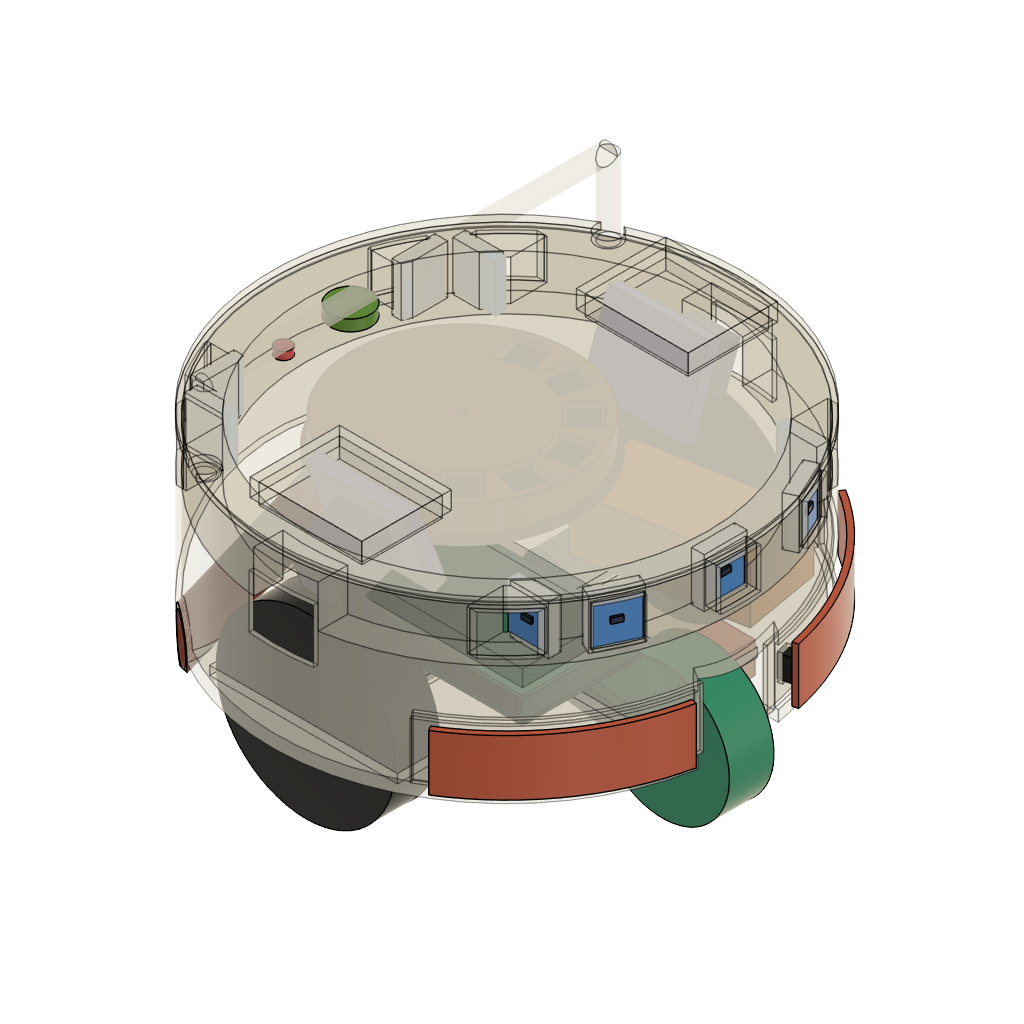
Theseus_V3_baseline (Autodesk Fusion 360 design; units mm, degrees)
Autodesk Fusion 360 part; units mm, degrees
(part 1 of 2)
sketch "Chassis shell sketch" plane through (0, 0, 0) normal (0, 0, 1) x (1, 0, 0) in component "Chassis"
  circle A0 centre (0, 0) radius 105
extrude "Chassis shell" add sketch "Chassis shell sketch" along normal blind 77 from surface at 35 makes body 1 in component "Chassis"
sketch "Cavity sketch" plane through (0, 0, 0) normal (0, 0, 1) x (1, 0, 0) in component "Chassis"
  circle A0 centre (0, 0) radius 103
extrude "Cavity" cut sketch "Cavity sketch" along normal blind 78 from surface at 39 bodies 1 in component "Chassis"
sketch "Rear chamfer sketch" plane through (0, 0, 0) normal (0, 1, 0) x (1, 0, 0) in component "Chassis"
  line L0 (-65, -35) -> (-112, -56.15)
  line L1 (-112, -56.15) -> (-112, -29)
  line L2 (-112, -29) -> (-65, -29)
  line L3 (-65, -29) -> (-65, -35)
extrude "Rear chamfer" cut sketch "Rear chamfer sketch" along normal blind 220 from surface at -110 bodies 1 in component "Chassis"
sketch "Wheel opening L sketch" plane through (0, 0, 0) normal (0, 0, 1) x (1, 0, 0) in component "Chassis"
  line L0 (-42, 69) -> (42, 69)
  line L1 (42, 69) -> (42, 91)
  line L2 (42, 91) -> (-42, 91)
  line L3 (-42, 91) -> (-42, 69)
extrude "Wheel opening L" cut sketch "Wheel opening L sketch" along normal blind 6 from surface at 34 bodies 1 in component "Chassis"
sketch "Motor and shaft slot L sketch" plane through (0, 0, 0) normal (0, 0, 1) x (1, 0, 0) in component "Chassis"
  line L0 (-10.5, 13.5) -> (10.5, 13.5)
  line L1 (10.5, 13.5) -> (10.5, 91)
  line L2 (10.5, 91) -> (-10.5, 91)
  line L3 (-10.5, 91) -> (-10.5, 13.5)
extrude "Motor and shaft slot L" cut sketch "Motor and shaft slot L sketch" along normal blind 6 from surface at 34 bodies 1 in component "Chassis"
sketch "Wheel opening R sketch" plane through (0, 0, 0) normal (0, 0, 1) x (1, 0, 0) in component "Chassis"
  line L0 (-42, -91) -> (42, -91)
  line L1 (42, -91) -> (42, -69)
  line L2 (42, -69) -> (-42, -69)
  line L3 (-42, -69) -> (-42, -91)
extrude "Wheel opening R" cut sketch "Wheel opening R sketch" along normal blind 6 from surface at 34 bodies 1 in component "Chassis"
sketch "Motor and shaft slot R sketch" plane through (0, 0, 0) normal (0, 0, 1) x (1, 0, 0) in component "Chassis"
  line L0 (-10.5, -91) -> (10.5, -91)
  line L1 (10.5, -91) -> (10.5, -13.5)
  line L2 (10.5, -13.5) -> (-10.5, -13.5)
  line L3 (-10.5, -13.5) -> (-10.5, -91)
extrude "Motor and shaft slot R" cut sketch "Motor and shaft slot R sketch" along normal blind 6 from surface at 34 bodies 1 in component "Chassis"
sketch "Omni bay 1 sketch" plane through (0, 0, 0) normal (0, 1, 0) x (1, 0, 0) in component "Chassis"
  line L0 (48.0005, -29.8229) -> (47.9302, -42.3229)
  arc A0 (47.9302, -42.3229) -> (110.9292, -42.6771) centre (79.4297, -42.5) ccw
  line L1 (110.9292, -42.6771) -> (110.9995, -30.1771)
  arc A1 (110.9995, -30.1771) -> (48.0005, -29.8229) centre (79.5, -30) ccw
extrude "Omni bay 1" cut sketch "Omni bay 1 sketch" along normal blind 36 from surface at -18 bodies 1 in component "Chassis"
sketch "Omni bay 2 sketch" plane through (0, 0, 0) normal (0, 1, 0) x (1, 0, 0) in component "Chassis"
  line L0 (49.2548, -33.4597) -> (45.5099, -45.9597)
  arc A0 (45.5099, -45.9597) -> (105.8596, -64.0403) centre (75.6848, -55) ccw
  line L1 (105.8596, -64.0403) -> (109.6046, -51.5403)
  arc A1 (109.6046, -51.5403) -> (49.2548, -33.4597) centre (79.4297, -42.5) ccw
extrude "Omni bay 2" cut sketch "Omni bay 2 sketch" along normal blind 36 from surface at -18 bodies 1 in component "Chassis"
sketch "Arm bay rest sketch" plane through (0, 0, 0) normal (0, 1, 0) x (1, 0, 0) in component "Chassis"
  line L0 (36.069, -43.9283) -> (80.569, -37.9283)
  arc A0 (80.569, -37.9283) -> (78.431, -22.0717) centre (79.5, -30) ccw
  line L1 (78.431, -22.0717) -> (33.931, -28.0717)
  arc A1 (33.931, -28.0717) -> (36.069, -43.9283) centre (35, -36) ccw
extrude "Arm bay rest" cut sketch "Arm bay rest sketch" along normal blind 36 from surface at -18 bodies 1 in component "Chassis"
sketch "Arm bay mid sketch" plane through (0, 0, 0) normal (0, 1, 0) x (1, 0, 0) in component "Chassis"
  line L0 (33.8419, -43.9157) -> (78.2717, -50.4157)
  arc A0 (78.2717, -50.4157) -> (80.5878, -34.5843) centre (79.4297, -42.5) ccw
  line L1 (80.5878, -34.5843) -> (36.1581, -28.0843)
  arc A1 (36.1581, -28.0843) -> (33.8419, -43.9157) centre (35, -36) ccw
extrude "Arm bay mid" cut sketch "Arm bay mid sketch" along normal blind 36 from surface at -18 bodies 1 in component "Chassis"
sketch "Arm bay compressed sketch" plane through (0, 0, 0) normal (0, 1, 0) x (1, 0, 0) in component "Chassis"
  line L0 (31.6149, -43.2485) -> (72.2997, -62.2485)
  arc A0 (72.2997, -62.2485) -> (79.0699, -47.7515) centre (75.6848, -55) ccw
  line L1 (79.0699, -47.7515) -> (38.3851, -28.7515)
  arc A1 (38.3851, -28.7515) -> (31.6149, -43.2485) centre (35, -36) ccw
extrude "Arm bay compressed" cut sketch "Arm bay compressed sketch" along normal blind 36 from surface at -18 bodies 1 in component "Chassis"
sketch "Floor port FP hole sketch" plane through (0, 0, 0) normal (0, 0, 1) x (1, 0, 0) in component "Chassis"
  line L0 (56.5, 21.5) -> (73.5, 21.5)
  line L1 (73.5, 21.5) -> (73.5, 38.5)
  line L2 (73.5, 38.5) -> (56.5, 38.5)
  line L3 (56.5, 38.5) -> (56.5, 21.5)
extrude "Floor port FP hole" cut sketch "Floor port FP hole sketch" along normal blind 6 from surface at 34 bodies 1 in component "Chassis"
sketch "Silver module SM hole sketch" plane through (0, 0, 0) normal (0, 0, 1) x (1, 0, 0) in component "Chassis"
  line L0 (-10.5, -11.5) -> (10.5, -11.5)
  line L1 (10.5, -11.5) -> (10.5, 11.5)
  line L2 (10.5, 11.5) -> (-10.5, 11.5)
  line L3 (-10.5, 11.5) -> (-10.5, -11.5)
extrude "Silver module SM hole" cut sketch "Silver module SM hole sketch" along normal blind 6 from surface at 34 bodies 1 in component "Chassis"
sketch "Chute hole tool B left sketch" plane through (0, 0, 0) normal (0, 0, 1) x (1, 0, 0) in component "Chassis"
  circle A0 centre (0, 0) radius 9
extrude "Chute hole tool B left" add sketch "Chute hole tool B left sketch" along normal blind 78.4275 separate body makes body 2 in component "Chassis"
move_body "Move1" bodies 2 to x (-0.977496, -0.210954, 0) y (-0.120664, 0.559121, 0.820259) z (-0.173037, 0.801799, -0.571993) at (-47.2943, 27.2943, 79.5) in component "Chassis"
combine "Combine1" operation cut target body 1 tool bodies 2 in component "Chassis"
sketch "Chute hole tool A right sketch" plane through (0, 0, 0) normal (0, 0, 1) x (1, 0, 0) in component "Chassis"
  circle A0 centre (0, 0) radius 9
extrude "Chute hole tool A right" add sketch "Chute hole tool A right sketch" along normal blind 78.4275 separate body makes body 3 in component "Chassis"
move_body "Move2" bodies 3 to x (0.977496, -0.210954, 0) y (-0.120664, -0.559121, 0.820259) z (-0.173037, -0.801799, -0.571993) at (-47.2943, -27.2943, 79.5) in component "Chassis"
combine "Combine2" operation cut target body 1 tool bodies 3 in component "Chassis"
sketch "ToF window F sketch" plane through (0, 0, 0) normal (0, 0, 1) x (1, 0, 0) in component "Chassis"
  line L0 (95, 9) -> (108, 9)
  line L1 (108, 9) -> (108, -9)
  line L2 (108, -9) -> (95, -9)
  line L3 (95, -9) -> (95, 9)
extrude "ToF window F" cut sketch "ToF window F sketch" along normal blind 18 from surface at 91 bodies 1 in component "Chassis"
sketch "ToF window FL sketch" plane through (0, 0, 0) normal (0, 0, 1) x (1, 0, 0) in component "Chassis"
  line L0 (85.9209, 49.996) -> (94.0777, 53.7995)
  line L1 (94.0777, 53.7995) -> (101.6848, 37.486)
  line L2 (101.6848, 37.486) -> (93.528, 33.6824)
  line L3 (93.528, 33.6824) -> (85.9209, 49.996)
extrude "ToF window FL" cut sketch "ToF window FL sketch" along normal blind 18 from surface at 91 bodies 1 in component "Chassis"
sketch "ToF window FR sketch" plane through (0, 0, 0) normal (0, 0, 1) x (1, 0, 0) in component "Chassis"
  line L0 (93.528, -33.6824) -> (101.6848, -37.486)
  line L1 (101.6848, -37.486) -> (94.0777, -53.7995)
  line L2 (94.0777, -53.7995) -> (85.9209, -49.996)
  line L3 (85.9209, -49.996) -> (93.528, -33.6824)
extrude "ToF window FR" cut sketch "ToF window FR sketch" along normal blind 18 from surface at 91 bodies 1 in component "Chassis"
sketch "ToF window SFL sketch" plane through (0, 0, 0) normal (0, 0, 1) x (1, 0, 0) in component "Chassis"
  line L0 (62.8, 60) -> (62.8, 80.6769)
  line L1 (62.8, 80.6769) -> (80.8, 80.6769)
  line L2 (80.8, 80.6769) -> (80.8, 60)
  line L3 (80.8, 60) -> (62.8, 60)
extrude "ToF window SFL" cut sketch "ToF window SFL sketch" along normal blind 18 from surface at 91 bodies 1 in component "Chassis"
sketch "ToF window SFR sketch" plane through (0, 0, 0) normal (0, 0, 1) x (1, 0, 0) in component "Chassis"
  line L0 (80.8, -60) -> (80.8, -80.6769)
  line L1 (80.8, -80.6769) -> (62.8, -80.6769)
  line L2 (62.8, -80.6769) -> (62.8, -60)
  line L3 (62.8, -60) -> (80.8, -60)
extrude "ToF window SFR" cut sketch "ToF window SFR sketch" along normal blind 18 from surface at 91 bodies 1 in component "Chassis"
sketch "ToF window SRL sketch" plane through (0, 0, 0) normal (0, 0, 1) x (1, 0, 0) in component "Chassis"
  line L0 (-80.8, 60) -> (-80.8, 80.6769)
  line L1 (-80.8, 80.6769) -> (-62.8, 80.6769)
  line L2 (-62.8, 80.6769) -> (-62.8, 60)
  line L3 (-62.8, 60) -> (-80.8, 60)
extrude "ToF window SRL" cut sketch "ToF window SRL sketch" along normal blind 18 from surface at 91 bodies 1 in component "Chassis"
sketch "ToF window SRR sketch" plane through (0, 0, 0) normal (0, 0, 1) x (1, 0, 0) in component "Chassis"
  line L0 (-62.8, -60) -> (-62.8, -80.6769)
  line L1 (-62.8, -80.6769) -> (-80.8, -80.6769)
  line L2 (-80.8, -80.6769) -> (-80.8, -60)
  line L3 (-80.8, -60) -> (-62.8, -60)
extrude "ToF window SRR" cut sketch "ToF window SRR sketch" along normal blind 18 from surface at 91 bodies 1 in component "Chassis"
sketch "ToF window RL sketch" plane through (0, 0, 0) normal (0, 0, 1) x (1, 0, 0) in component "Chassis"
  line L0 (-84, 36) -> (-98.1784, 36)
  line L1 (-98.1784, 36) -> (-98.1784, 54)
  line L2 (-98.1784, 54) -> (-84, 54)
  line L3 (-84, 54) -> (-84, 36)
extrude "ToF window RL" cut sketch "ToF window RL sketch" along normal blind 18 from surface at 91 bodies 1 in component "Chassis"
sketch "ToF window RR sketch" plane through (0, 0, 0) normal (0, 0, 1) x (1, 0, 0) in component "Chassis"
  line L0 (-84, -54) -> (-98.1784, -54)
  line L1 (-98.1784, -54) -> (-98.1784, -36)
  line L2 (-98.1784, -36) -> (-84, -36)
  line L3 (-84, -36) -> (-84, -54)
extrude "ToF window RR" cut sketch "ToF window RR sketch" along normal blind 18 from surface at 91 bodies 1 in component "Chassis"
sketch "Camera window L sketch" plane through (0, 0, 0) normal (0, 1, 0) x (1, 0, 0) in component "Chassis"
  line L0 (-10.9288, -74) -> (17.0712, -74)
  line L1 (17.0712, -74) -> (17.0712, -98)
  line L2 (17.0712, -98) -> (-10.9288, -98)
  line L3 (-10.9288, -98) -> (-10.9288, -74)
extrude "Camera window L" cut sketch "Camera window L sketch" along normal blind 19 from surface at 89 bodies 1 in component "Chassis"
sketch "Camera window R sketch" plane through (0, 0, 0) normal (0, 1, 0) x (1, 0, 0) in component "Chassis"
  line L0 (-10.9288, -74) -> (17.0712, -74)
  line L1 (17.0712, -74) -> (17.0712, -98)
  line L2 (17.0712, -98) -> (-10.9288, -98)
  line L3 (-10.9288, -98) -> (-10.9288, -74)
extrude "Camera window R" cut sketch "Camera window R sketch" along normal blind 19 from surface at -108 bodies 1 in component "Chassis"
sketch "Bumper recess L sketch" plane through (0, 0, 0) normal (0, 0, 1) x (1, 0, 0) in component "Chassis"
  arc A0 (106.949, 15.0307) -> (50.7029, 95.3583) centre (0, 0) ccw
  line L0 (50.7029, 95.3583) -> (48.5903, 91.3851)
  arc A1 (102.4927, 14.4044) -> (48.5903, 91.3851) centre (0, 0) ccw
  line L1 (102.4927, 14.4044) -> (106.949, 15.0307)
extrude "Bumper recess L" cut sketch "Bumper recess L sketch" along normal blind 25 from surface at 40 bodies 1 in component "Chassis"
sketch "Bumper recess wall L sketch" plane through (0, 0, 0) normal (0, 0, 1) x (1, 0, 0) in component "Chassis"
  arc A0 (102.1957, 14.3627) -> (48.4495, 91.1202) centre (0, 0) ccw
  line L0 (48.4495, 91.1202) -> (47.6514, 89.6192)
  arc A1 (100.5122, 14.1261) -> (47.6514, 89.6192) centre (0, 0) ccw
  line L1 (100.5122, 14.1261) -> (102.1957, 14.3627)
extrude "Bumper recess wall L" add sketch "Bumper recess wall L sketch" along normal blind 27 from surface at 39 bodies 1 in component "Chassis"
sketch "Bumper switch pocket L sketch" plane through (0, 0, 0) normal (0, 0, 1) x (1, 0, 0) in component "Chassis"
  line L0 (98.18, 21.6448) -> (101.576, 22.4916)
  line L1 (101.576, 22.4916) -> (100.2455, 27.8282)
  line L2 (100.2455, 27.8282) -> (96.8494, 26.9815)
  line L3 (96.8494, 26.9815) -> (98.18, 21.6448)
extrude "Bumper switch pocket L" cut sketch "Bumper switch pocket L sketch" along normal blind 12 from surface at 46.5 bodies 1 in component "Chassis"
sketch "Bumper recess R sketch" plane through (0, 0, 0) normal (0, 0, 1) x (1, 0, 0) in component "Chassis"
  arc A0 (50.7029, -95.3583) -> (106.949, -15.0307) centre (0, 0) ccw
  line L0 (106.949, -15.0307) -> (102.4927, -14.4044)
  arc A1 (48.5903, -91.3851) -> (102.4927, -14.4044) centre (0, 0) ccw
  line L1 (48.5903, -91.3851) -> (50.7029, -95.3583)
extrude "Bumper recess R" cut sketch "Bumper recess R sketch" along normal blind 25 from surface at 40 bodies 1 in component "Chassis"
sketch "Bumper recess wall R sketch" plane through (0, 0, 0) normal (0, 0, 1) x (1, 0, 0) in component "Chassis"
  arc A0 (48.4495, -91.1202) -> (102.1957, -14.3627) centre (0, 0) ccw
  line L0 (102.1957, -14.3627) -> (100.5122, -14.1261)
  arc A1 (47.6514, -89.6192) -> (100.5122, -14.1261) centre (0, 0) ccw
  line L1 (47.6514, -89.6192) -> (48.4495, -91.1202)
extrude "Bumper recess wall R" add sketch "Bumper recess wall R sketch" along normal blind 27 from surface at 39 bodies 1 in component "Chassis"
sketch "Bumper switch pocket R sketch" plane through (0, 0, 0) normal (0, 0, 1) x (1, 0, 0) in component "Chassis"
  line L0 (96.8494, -26.9815) -> (100.2455, -27.8282)
  line L1 (100.2455, -27.8282) -> (101.576, -22.4916)
  line L2 (101.576, -22.4916) -> (98.18, -21.6448)
  line L3 (98.18, -21.6448) -> (96.8494, -26.9815)
extrude "Bumper switch pocket R" cut sketch "Bumper switch pocket R sketch" along normal blind 12 from surface at 46.5 bodies 1 in component "Chassis"
sketch "Handle post L sketch" plane through (0, 0, 0) normal (0, 0, 1) x (1, 0, 0) in component "Chassis"
  circle A0 centre (-45, 90.4) radius 4
extrude "Handle post L" add sketch "Handle post L sketch" along normal blind 34.5 from surface at 111.5 bodies 1 in component "Chassis"
sketch "Handle post R sketch" plane through (0, 0, 0) normal (0, 0, 1) x (1, 0, 0) in component "Chassis"
  circle A0 centre (-45, -90.4) radius 4
extrude "Handle post R" add sketch "Handle post R sketch" along normal blind 34.5 from surface at 111.5 bodies 1 in component "Chassis"
sketch "Handle bar sketch" plane through (0, 0, 0) normal (0, 1, 0) x (1, 0, 0) in component "Chassis"
  circle A0 centre (-45, -146) radius 4
extrude "Handle bar" add sketch "Handle bar sketch" along normal blind 180.8 from surface at -90.4 bodies 1 in component "Chassis"
sketch "Wheel L sketch" plane through (0, 0, 0) normal (0, 1, 0) x (1, 0, 0) in component "Wheel L"
  circle A0 centre (0, -40) radius 40
extrude "Wheel L" add sketch "Wheel L sketch" along normal blind 20 from surface at 70 separate body makes body 4 in component "Wheel L"
sketch "Shaft bore sketch" plane through (0, 0, 0) normal (0, 1, 0) x (1, 0, 0) in component "Wheel L"
  circle A0 centre (0, -40) radius 1.5
extrude "Shaft bore" cut sketch "Shaft bore sketch" along normal blind 22 from surface at 69 bodies 4 in component "Wheel L"
sketch "Encoder L sketch" plane through (0, 0, 0) normal (0, 1, 0) x (1, 0, 0) in component "Motor L"
  circle A0 centre (0, -40) radius 9
extrude "Encoder L" add sketch "Encoder L sketch" along normal blind 3 from surface at 14 separate body makes body 5 in component "Motor L"
sketch "Gearmotor L sketch" plane through (0, 0, 0) normal (0, 1, 0) x (1, 0, 0) in component "Motor L"
  circle A0 centre (0, -40) radius 10
extrude "Gearmotor L" add sketch "Gearmotor L sketch" along normal blind 44 from surface at 17 separate body makes body 6 in component "Motor L"
sketch "Motor shaft L sketch" plane through (0, 0, 0) normal (0, 1, 0) x (1, 0, 0) in component "Motor L"
  circle A0 centre (0, -40) radius 1.5
extrude "Motor shaft L" add sketch "Motor shaft L sketch" along normal blind 19 from surface at 61 separate body makes body 7 in component "Motor L"
sketch "Wheel R sketch" plane through (0, 0, 0) normal (0, 1, 0) x (1, 0, 0) in component "Wheel R"
  circle A0 centre (0, -40) radius 40
extrude "Wheel R" add sketch "Wheel R sketch" along normal blind 20 from surface at -90 separate body makes body 8 in component "Wheel R"
sketch "Shaft bore sketch (2)" plane through (0, 0, 0) normal (0, 1, 0) x (1, 0, 0) in component "Wheel R"
  circle A0 centre (0, -40) radius 1.5
extrude "Shaft bore'" cut sketch "Shaft bore sketch (2)" along normal blind 22 from surface at -91 bodies 8 in component "Wheel R"
sketch "Encoder R sketch" plane through (0, 0, 0) normal (0, 1, 0) x (1, 0, 0) in component "Motor R"
  circle A0 centre (0, -40) radius 9
extrude "Encoder R" add sketch "Encoder R sketch" along normal blind 3 from surface at -17 separate body makes body 9 in component "Motor R"
sketch "Gearmotor R sketch" plane through (0, 0, 0) normal (0, 1, 0) x (1, 0, 0) in component "Motor R"
  circle A0 centre (0, -40) radius 10
extrude "Gearmotor R" add sketch "Gearmotor R sketch" along normal blind 44 from surface at -61 separate body makes body 10 in component "Motor R"
sketch "Motor shaft R sketch" plane through (0, 0, 0) normal (0, 1, 0) x (1, 0, 0) in component "Motor R"
  circle A0 centre (0, -40) radius 1.5
extrude "Motor shaft R" add sketch "Motor shaft R sketch" along normal blind 19 from surface at -80 separate body makes body 11 in component "Motor R"
sketch "Omni wheel sketch" plane through (0, 0, 0) normal (0, 1, 0) x (1, 0, 0) in component "Omni wheel"
  circle A0 centre (79.5, -30) radius 30
extrude "Omni wheel" add sketch "Omni wheel sketch" along normal blind 20 from surface at -10 separate body makes body 12 in component "Omni wheel"
sketch "Omni hub sketch" plane through (0, 0, 0) normal (0, 1, 0) x (1, 0, 0) in component "Omni wheel"
  circle A0 centre (79.5, -30) radius 10
extrude "Omni hub" add sketch "Omni hub sketch" along normal blind 22 from surface at -11 bodies 12 in component "Omni wheel"
sketch "Axle bore sketch" plane through (0, 0, 0) normal (0, 1, 0) x (1, 0, 0) in component "Omni wheel"
  circle A0 centre (79.5, -30) radius 2
extrude "Axle bore" cut sketch "Axle bore sketch" along normal blind 24 from surface at -12 bodies 12 in component "Omni wheel"
sketch "Arm plate L sketch" plane through (0, 0, 0) normal (0, 1, 0) x (1, 0, 0) in component "Omni arm"
  line L0 (35.7349, -41.4507) -> (80.2349, -35.4507)
  arc A0 (80.2349, -35.4507) -> (78.7651, -24.5493) centre (79.5, -30) ccw
  line L1 (78.7651, -24.5493) -> (34.2651, -30.5493)
  arc A1 (34.2651, -30.5493) -> (35.7349, -41.4507) centre (35, -36) ccw
extrude "Arm plate L" add sketch "Arm plate L sketch" along normal blind 4 from surface at 11 separate body makes body 13 in component "Omni arm"
sketch "Pivot hole L sketch" plane through (0, 0, 0) normal (0, 1, 0) x (1, 0, 0) in component "Omni arm"
  circle A0 centre (35, -36) radius 2
extrude "Pivot hole L" cut sketch "Pivot hole L sketch" along normal blind 6 from surface at 10 bodies 13 in component "Omni arm"
sketch "Axle hole L sketch" plane through (0, 0, 0) normal (0, 1, 0) x (1, 0, 0) in component "Omni arm"
  circle A0 centre (79.5, -30) radius 2
extrude "Axle hole L" cut sketch "Axle hole L sketch" along normal blind 6 from surface at 10 bodies 13 in component "Omni arm"
sketch "Arm plate R sketch" plane through (0, 0, 0) normal (0, 1, 0) x (1, 0, 0) in component "Omni arm"
  line L0 (35.7349, -41.4507) -> (80.2349, -35.4507)
  arc A0 (80.2349, -35.4507) -> (78.7651, -24.5493) centre (79.5, -30) ccw
  line L1 (78.7651, -24.5493) -> (34.2651, -30.5493)
  arc A1 (34.2651, -30.5493) -> (35.7349, -41.4507) centre (35, -36) ccw
extrude "Arm plate R" add sketch "Arm plate R sketch" along normal blind 4 from surface at -15 separate body makes body 14 in component "Omni arm"
sketch "Pivot hole R sketch" plane through (0, 0, 0) normal (0, 1, 0) x (1, 0, 0) in component "Omni arm"
  circle A0 centre (35, -36) radius 2
extrude "Pivot hole R" cut sketch "Pivot hole R sketch" along normal blind 6 from surface at -16 bodies 14 in component "Omni arm"
sketch "Axle hole R sketch" plane through (0, 0, 0) normal (0, 1, 0) x (1, 0, 0) in component "Omni arm"
  circle A0 centre (79.5, -30) radius 2
extrude "Axle hole R" cut sketch "Axle hole R sketch" along normal blind 6 from surface at -16 bodies 14 in component "Omni arm"
sketch "Pivot pin sketch" plane through (0, 0, 0) normal (0, 1, 0) x (1, 0, 0) in component "Omni pins"
  circle A0 centre (35, -36) radius 2
extrude "Pivot pin" add sketch "Pivot pin sketch" along normal blind 34 from surface at -17 separate body makes body 15 in component "Omni pins"
sketch "Axle pin sketch" plane through (0, 0, 0) normal (0, 1, 0) x (1, 0, 0) in component "Omni pins"
  circle A0 centre (79.5, -30) radius 2
extrude "Axle pin" add sketch "Axle pin sketch" along normal blind 30 from surface at -15 separate body makes body 16 in component "Omni pins"
sketch "Rear nub sketch" plane through (0, 0, 0) normal (0, 0, 1) x (1, 0, 0) in component "Rear nub"
  circle A0 centre (-80, 0) radius 4
extrude "Rear nub" add sketch "Rear nub sketch" along normal blind 26 from surface at 20 separate body makes body 17 in component "Rear nub"
sketch "Seat on chamfer sketch" plane through (0, 0, 0) normal (0, 1, 0) x (1, 0, 0) in component "Rear nub"
  line L0 (-65, -35) -> (-112, -56.15)
  line L1 (-112, -56.15) -> (-112, -70)
  line L2 (-112, -70) -> (-65, -70)
  line L3 (-65, -70) -> (-65, -35)
extrude "Seat on chamfer" cut sketch "Seat on chamfer sketch" along normal blind 20 from surface at -10 bodies 17 in component "Rear nub"
sketch "Bumper plate L sketch" plane through (0, 0, 0) normal (0, 0, 1) x (1, 0, 0) in component "Bumper L"
  arc A0 (107.5962, 22.8703) -> (58.2911, 93.2853) centre (0, 0) ccw
  line L0 (58.2911, 93.2853) -> (56.9663, 91.1652)
  arc A1 (105.1509, 22.3505) -> (56.9663, 91.1652) centre (0, 0) ccw
  line L1 (105.1509, 22.3505) -> (107.5962, 22.8703)
extrude "Bumper plate L" add sketch "Bumper plate L sketch" along normal blind 25 from surface at 40 separate body makes body 18 in component "Bumper L"
sketch "Microswitch L sketch" plane through (0, 0, 0) normal (0, 0, 1) x (1, 0, 0) in component "Bumper switch L"
  line L0 (98.5442, 22.2509) -> (104.8511, 23.8234)
  line L1 (104.8511, 23.8234) -> (103.7625, 28.1898)
  line L2 (103.7625, 28.1898) -> (97.4555, 26.6173)
  line L3 (97.4555, 26.6173) -> (98.5442, 22.2509)
extrude "Microswitch L" add sketch "Microswitch L sketch" along normal blind 10 from surface at 47.5 separate body makes body 19 in component "Bumper switch L"
sketch "Bumper plate R sketch" plane through (0, 0, 0) normal (0, 0, 1) x (1, 0, 0) in component "Bumper R"
  arc A0 (58.2911, -93.2853) -> (107.5962, -22.8703) centre (0, 0) ccw
  line L0 (107.5962, -22.8703) -> (105.1509, -22.3505)
  arc A1 (56.9663, -91.1652) -> (105.1509, -22.3505) centre (0, 0) ccw
  line L1 (56.9663, -91.1652) -> (58.2911, -93.2853)
extrude "Bumper plate R" add sketch "Bumper plate R sketch" along normal blind 25 from surface at 40 separate body makes body 20 in component "Bumper R"
sketch "Microswitch R sketch" plane through (0, 0, 0) normal (0, 0, 1) x (1, 0, 0) in component "Bumper switch R"
  line L0 (97.4555, -26.6173) -> (103.7625, -28.1898)
  line L1 (103.7625, -28.1898) -> (104.8511, -23.8234)
  line L2 (104.8511, -23.8234) -> (98.5442, -22.2509)
  line L3 (98.5442, -22.2509) -> (97.4555, -26.6173)
extrude "Microswitch R" add sketch "Microswitch R sketch" along normal blind 10 from surface at 47.5 separate body makes body 21 in component "Bumper switch R"
sketch "ToF ring sketch" plane through (0, 0, 0) normal (0, 0, 1) x (1, 0, 0) in component "ToF ring"
  circle A0 centre (0, 0) radius 103
  circle A1 centre (0, 0) radius 90
extrude "ToF ring" add sketch "ToF ring sketch" along normal blind 24.5 from surface at 87 separate body makes body 22 in component "ToF ring"
sketch "Pocket F sketch" plane through (0, 0, 0) normal (0, 0, 1) x (1, 0, 0) in component "ToF ring"
  line L0 (92.15, 9.6) -> (97.85, 9.6)
  line L1 (97.85, 9.6) -> (97.85, -9.6)
  line L2 (97.85, -9.6) -> (92.15, -9.6)
  line L3 (92.15, -9.6) -> (92.15, 9.6)
extrude "Pocket F" cut sketch "Pocket F sketch" along normal blind 22 from surface at 89 bodies 22 in component "ToF ring"
sketch "Beam F sketch" plane through (0, 0, 0) normal (0, 0, 1) x (1, 0, 0) in component "ToF ring"
  line L0 (95, 9) -> (108, 9)
  line L1 (108, 9) -> (108, -9)
  line L2 (108, -9) -> (95, -9)
  line L3 (95, -9) -> (95, 9)
extrude "Beam F" cut sketch "Beam F sketch" along normal blind 18 from surface at 91 bodies 22 in component "ToF ring"
sketch "Pocket FL sketch" plane through (0, 0, 0) normal (0, 0, 1) x (1, 0, 0) in component "ToF ring"
  line L0 (83.0844, 49.3353) -> (88.2503, 51.7442)
  line L1 (88.2503, 51.7442) -> (96.3646, 34.3431)
  line L2 (96.3646, 34.3431) -> (91.1986, 31.9342)
  line L3 (91.1986, 31.9342) -> (83.0844, 49.3353)
extrude "Pocket FL" cut sketch "Pocket FL sketch" along normal blind 22 from surface at 89 bodies 22 in component "ToF ring"
sketch "Beam FL sketch" plane through (0, 0, 0) normal (0, 0, 1) x (1, 0, 0) in component "ToF ring"
  line L0 (85.9209, 49.996) -> (94.0777, 53.7995)
  line L1 (94.0777, 53.7995) -> (101.6848, 37.486)
  line L2 (101.6848, 37.486) -> (93.528, 33.6824)
  line L3 (93.528, 33.6824) -> (85.9209, 49.996)
extrude "Beam FL" cut sketch "Beam FL sketch" along normal blind 18 from surface at 91 bodies 22 in component "ToF ring"
sketch "Pocket FR sketch" plane through (0, 0, 0) normal (0, 0, 1) x (1, 0, 0) in component "ToF ring"
  line L0 (91.1986, -31.9342) -> (96.3646, -34.3431)
  line L1 (96.3646, -34.3431) -> (88.2503, -51.7442)
  line L2 (88.2503, -51.7442) -> (83.0844, -49.3353)
  line L3 (83.0844, -49.3353) -> (91.1986, -31.9342)
extrude "Pocket FR" cut sketch "Pocket FR sketch" along normal blind 22 from surface at 89 bodies 22 in component "ToF ring"
sketch "Beam FR sketch" plane through (0, 0, 0) normal (0, 0, 1) x (1, 0, 0) in component "ToF ring"
  line L0 (93.528, -33.6824) -> (101.6848, -37.486)
  line L1 (101.6848, -37.486) -> (94.0777, -53.7995)
  line L2 (94.0777, -53.7995) -> (85.9209, -49.996)
  line L3 (85.9209, -49.996) -> (93.528, -33.6824)
extrude "Beam FR" cut sketch "Beam FR sketch" along normal blind 18 from surface at 91 bodies 22 in component "ToF ring"
sketch "Pocket SFL sketch" plane through (0, 0, 0) normal (0, 0, 1) x (1, 0, 0) in component "ToF ring"
  line L0 (62.2, 57.15) -> (62.2, 62.85)
  line L1 (62.2, 62.85) -> (81.4, 62.85)
  line L2 (81.4, 62.85) -> (81.4, 57.15)
  line L3 (81.4, 57.15) -> (62.2, 57.15)
extrude "Pocket SFL" cut sketch "Pocket SFL sketch" along normal blind 22 from surface at 89 bodies 22 in component "ToF ring"
sketch "Beam SFL sketch" plane through (0, 0, 0) normal (0, 0, 1) x (1, 0, 0) in component "ToF ring"
  line L0 (62.8, 60) -> (62.8, 80.6769)
  line L1 (62.8, 80.6769) -> (80.8, 80.6769)
  line L2 (80.8, 80.6769) -> (80.8, 60)
  line L3 (80.8, 60) -> (62.8, 60)
extrude "Beam SFL" cut sketch "Beam SFL sketch" along normal blind 18 from surface at 91 bodies 22 in component "ToF ring"
sketch "Pocket SFR sketch" plane through (0, 0, 0) normal (0, 0, 1) x (1, 0, 0) in component "ToF ring"
  line L0 (81.4, -57.15) -> (81.4, -62.85)
  line L1 (81.4, -62.85) -> (62.2, -62.85)
  line L2 (62.2, -62.85) -> (62.2, -57.15)
  line L3 (62.2, -57.15) -> (81.4, -57.15)
extrude "Pocket SFR" cut sketch "Pocket SFR sketch" along normal blind 22 from surface at 89 bodies 22 in component "ToF ring"
sketch "Beam SFR sketch" plane through (0, 0, 0) normal (0, 0, 1) x (1, 0, 0) in component "ToF ring"
  line L0 (80.8, -60) -> (80.8, -80.6769)
  line L1 (80.8, -80.6769) -> (62.8, -80.6769)
  line L2 (62.8, -80.6769) -> (62.8, -60)
  line L3 (62.8, -60) -> (80.8, -60)
extrude "Beam SFR" cut sketch "Beam SFR sketch" along normal blind 18 from surface at 91 bodies 22 in component "ToF ring"
sketch "Pocket SRL sketch" plane through (0, 0, 0) normal (0, 0, 1) x (1, 0, 0) in component "ToF ring"
  line L0 (-81.4, 57.15) -> (-81.4, 62.85)
  line L1 (-81.4, 62.85) -> (-62.2, 62.85)
  line L2 (-62.2, 62.85) -> (-62.2, 57.15)
  line L3 (-62.2, 57.15) -> (-81.4, 57.15)
extrude "Pocket SRL" cut sketch "Pocket SRL sketch" along normal blind 22 from surface at 89 bodies 22 in component "ToF ring"
sketch "Beam SRL sketch" plane through (0, 0, 0) normal (0, 0, 1) x (1, 0, 0) in component "ToF ring"
  line L0 (-80.8, 60) -> (-80.8, 80.6769)
  line L1 (-80.8, 80.6769) -> (-62.8, 80.6769)
  line L2 (-62.8, 80.6769) -> (-62.8, 60)
  line L3 (-62.8, 60) -> (-80.8, 60)
extrude "Beam SRL" cut sketch "Beam SRL sketch" along normal blind 18 from surface at 91 bodies 22 in component "ToF ring"
sketch "Pocket SRR sketch" plane through (0, 0, 0) normal (0, 0, 1) x (1, 0, 0) in component "ToF ring"
  line L0 (-62.2, -57.15) -> (-62.2, -62.85)
  line L1 (-62.2, -62.85) -> (-81.4, -62.85)
  line L2 (-81.4, -62.85) -> (-81.4, -57.15)
  line L3 (-81.4, -57.15) -> (-62.2, -57.15)
extrude "Pocket SRR" cut sketch "Pocket SRR sketch" along normal blind 22 from surface at 89 bodies 22 in component "ToF ring"
sketch "Beam SRR sketch" plane through (0, 0, 0) normal (0, 0, 1) x (1, 0, 0) in component "ToF ring"
  line L0 (-62.8, -60) -> (-62.8, -80.6769)
  line L1 (-62.8, -80.6769) -> (-80.8, -80.6769)
  line L2 (-80.8, -80.6769) -> (-80.8, -60)
  line L3 (-80.8, -60) -> (-62.8, -60)
extrude "Beam SRR" cut sketch "Beam SRR sketch" along normal blind 18 from surface at 91 bodies 22 in component "ToF ring"
sketch "Pocket RL sketch" plane through (0, 0, 0) normal (0, 0, 1) x (1, 0, 0) in component "ToF ring"
  line L0 (-81.15, 35.4) -> (-86.85, 35.4)
  line L1 (-86.85, 35.4) -> (-86.85, 54.6)
  line L2 (-86.85, 54.6) -> (-81.15, 54.6)
  line L3 (-81.15, 54.6) -> (-81.15, 35.4)
extrude "Pocket RL" cut sketch "Pocket RL sketch" along normal blind 22 from surface at 89 bodies 22 in component "ToF ring"
sketch "Beam RL sketch" plane through (0, 0, 0) normal (0, 0, 1) x (1, 0, 0) in component "ToF ring"
  line L0 (-84, 36) -> (-98.1784, 36)
  line L1 (-98.1784, 36) -> (-98.1784, 54)
  line L2 (-98.1784, 54) -> (-84, 54)
  line L3 (-84, 54) -> (-84, 36)
extrude "Beam RL" cut sketch "Beam RL sketch" along normal blind 18 from surface at 91 bodies 22 in component "ToF ring"
sketch "Pocket RR sketch" plane through (0, 0, 0) normal (0, 0, 1) x (1, 0, 0) in component "ToF ring"
  line L0 (-81.15, -54.6) -> (-86.85, -54.6)
  line L1 (-86.85, -54.6) -> (-86.85, -35.4)
  line L2 (-86.85, -35.4) -> (-81.15, -35.4)
  line L3 (-81.15, -35.4) -> (-81.15, -54.6)
extrude "Pocket RR" cut sketch "Pocket RR sketch" along normal blind 22 from surface at 89 bodies 22 in component "ToF ring"
sketch "Beam RR sketch" plane through (0, 0, 0) normal (0, 0, 1) x (1, 0, 0) in component "ToF ring"
  line L0 (-84, -54) -> (-98.1784, -54)
  line L1 (-98.1784, -54) -> (-98.1784, -36)
  line L2 (-98.1784, -36) -> (-84, -36)
  line L3 (-84, -36) -> (-84, -54)
extrude "Beam RR" cut sketch "Beam RR sketch" along normal blind 18 from surface at 91 bodies 22 in component "ToF ring"
sketch "Camera window L sketch (2)" plane through (0, 0, 0) normal (0, 1, 0) x (1, 0, 0) in component "ToF ring"
  line L0 (-10.9288, -86) -> (17.0712, -86)
  line L1 (17.0712, -86) -> (17.0712, -106)
  line L2 (17.0712, -106) -> (-10.9288, -106)
  line L3 (-10.9288, -106) -> (-10.9288, -86)
extrude "Camera window L'" cut sketch "Camera window L sketch (2)" along normal blind 24 from surface at 84 bodies 22 in component "ToF ring"
sketch "Camera window R sketch (2)" plane through (0, 0, 0) normal (0, 1, 0) x (1, 0, 0) in component "ToF ring"
  line L0 (-10.9288, -86) -> (17.0712, -86)
  line L1 (17.0712, -86) -> (17.0712, -106)
  line L2 (17.0712, -106) -> (-10.9288, -106)
  line L3 (-10.9288, -106) -> (-10.9288, -86)
extrude "Camera window R'" cut sketch "Camera window R sketch (2)" along normal blind 24 from surface at -108 bodies 22 in component "ToF ring"
sketch "VL53L0X module F sketch" plane through (0, 0, 0) normal (0, 0, 1) x (1, 0, 0) in component "ToF F"
  line L0 (92.75, -9) -> (97.25, -9)
  line L1 (97.25, -9) -> (97.25, 9)
  line L2 (97.25, 9) -> (92.75, 9)
  line L3 (92.75, 9) -> (92.75, -9)
extrude "VL53L0X module F" add sketch "VL53L0X module F sketch" along normal blind 21 from surface at 89.5 separate body makes body 23 in component "ToF F"
sketch "VL53L0X chip F sketch" plane through (0, 0, 0) normal (0, 0, 1) x (1, 0, 0) in component "ToF F"
  line L0 (97.25, -2.2) -> (98.25, -2.2)
  line L1 (98.25, -2.2) -> (98.25, 2.2)
  line L2 (98.25, 2.2) -> (97.25, 2.2)
  line L3 (97.25, 2.2) -> (97.25, -2.2)
extrude "VL53L0X chip F" add sketch "VL53L0X chip F sketch" along normal blind 2.4 from surface at 98.8 separate body makes body 24 in component "ToF F"
sketch "VL53L0X module FL sketch" plane through (0, 0, 0) normal (0, 0, 1) x (1, 0, 0) in component "ToF FL"
  line L0 (91.4888, 32.7315) -> (95.5672, 34.6333)
  line L1 (95.5672, 34.6333) -> (87.9601, 50.9469)
  line L2 (87.9601, 50.9469) -> (83.8817, 49.0451)
  line L3 (83.8817, 49.0451) -> (91.4888, 32.7315)
extrude "VL53L0X module FL" add sketch "VL53L0X module FL sketch" along normal blind 21 from surface at 89.5 separate body makes body 25 in component "ToF FL"
sketch "VL53L0X chip FL sketch" plane through (0, 0, 0) normal (0, 0, 1) x (1, 0, 0) in component "ToF FL"
  line L0 (92.6934, 40.7962) -> (93.5997, 41.2188)
  line L1 (93.5997, 41.2188) -> (91.7402, 45.2066)
  line L2 (91.7402, 45.2066) -> (90.8339, 44.784)
  line L3 (90.8339, 44.784) -> (92.6934, 40.7962)
extrude "VL53L0X chip FL" add sketch "VL53L0X chip FL sketch" along normal blind 2.4 from surface at 98.8 separate body makes body 26 in component "ToF FL"
sketch "VL53L0X module FR sketch" plane through (0, 0, 0) normal (0, 0, 1) x (1, 0, 0) in component "ToF FR"
  line L0 (83.8817, -49.0451) -> (87.9601, -50.9469)
  line L1 (87.9601, -50.9469) -> (95.5672, -34.6333)
  line L2 (95.5672, -34.6333) -> (91.4888, -32.7315)
  line L3 (91.4888, -32.7315) -> (83.8817, -49.0451)
extrude "VL53L0X module FR" add sketch "VL53L0X module FR sketch" along normal blind 21 from surface at 89.5 separate body makes body 27 in component "ToF FR"
sketch "VL53L0X chip FR sketch" plane through (0, 0, 0) normal (0, 0, 1) x (1, 0, 0) in component "ToF FR"
  line L0 (90.8339, -44.784) -> (91.7402, -45.2066)
  line L1 (91.7402, -45.2066) -> (93.5997, -41.2188)
  line L2 (93.5997, -41.2188) -> (92.6934, -40.7962)
  line L3 (92.6934, -40.7962) -> (90.8339, -44.784)
extrude "VL53L0X chip FR" add sketch "VL53L0X chip FR sketch" along normal blind 2.4 from surface at 98.8 separate body makes body 28 in component "ToF FR"
sketch "VL53L0X module SFL sketch" plane through (0, 0, 0) normal (0, 0, 1) x (1, 0, 0) in component "ToF SFL"
  line L0 (80.8, 57.75) -> (80.8, 62.25)
  line L1 (80.8, 62.25) -> (62.8, 62.25)
  line L2 (62.8, 62.25) -> (62.8, 57.75)
  line L3 (62.8, 57.75) -> (80.8, 57.75)
extrude "VL53L0X module SFL" add sketch "VL53L0X module SFL sketch" along normal blind 21 from surface at 89.5 separate body makes body 29 in component "ToF SFL"
sketch "VL53L0X chip SFL sketch" plane through (0, 0, 0) normal (0, 0, 1) x (1, 0, 0) in component "ToF SFL"
  line L0 (74, 62.25) -> (74, 63.25)
  line L1 (74, 63.25) -> (69.6, 63.25)
  line L2 (69.6, 63.25) -> (69.6, 62.25)
  line L3 (69.6, 62.25) -> (74, 62.25)
extrude "VL53L0X chip SFL" add sketch "VL53L0X chip SFL sketch" along normal blind 2.4 from surface at 98.8 separate body makes body 30 in component "ToF SFL"
sketch "VL53L0X module SFR sketch" plane through (0, 0, 0) normal (0, 0, 1) x (1, 0, 0) in component "ToF SFR"
  line L0 (62.8, -57.75) -> (62.8, -62.25)
  line L1 (62.8, -62.25) -> (80.8, -62.25)
  line L2 (80.8, -62.25) -> (80.8, -57.75)
  line L3 (80.8, -57.75) -> (62.8, -57.75)
extrude "VL53L0X module SFR" add sketch "VL53L0X module SFR sketch" along normal blind 21 from surface at 89.5 separate body makes body 31 in component "ToF SFR"
sketch "VL53L0X chip SFR sketch" plane through (0, 0, 0) normal (0, 0, 1) x (1, 0, 0) in component "ToF SFR"
  line L0 (69.6, -62.25) -> (69.6, -63.25)
  line L1 (69.6, -63.25) -> (74, -63.25)
  line L2 (74, -63.25) -> (74, -62.25)
  line L3 (74, -62.25) -> (69.6, -62.25)
extrude "VL53L0X chip SFR" add sketch "VL53L0X chip SFR sketch" along normal blind 2.4 from surface at 98.8 separate body makes body 32 in component "ToF SFR"
sketch "VL53L0X module SRL sketch" plane through (0, 0, 0) normal (0, 0, 1) x (1, 0, 0) in component "ToF SRL"
  line L0 (-62.8, 57.75) -> (-62.8, 62.25)
  line L1 (-62.8, 62.25) -> (-80.8, 62.25)
  line L2 (-80.8, 62.25) -> (-80.8, 57.75)
  line L3 (-80.8, 57.75) -> (-62.8, 57.75)
extrude "VL53L0X module SRL" add sketch "VL53L0X module SRL sketch" along normal blind 21 from surface at 89.5 separate body makes body 33 in component "ToF SRL"
sketch "VL53L0X chip SRL sketch" plane through (0, 0, 0) normal (0, 0, 1) x (1, 0, 0) in component "ToF SRL"
  line L0 (-69.6, 62.25) -> (-69.6, 63.25)
  line L1 (-69.6, 63.25) -> (-74, 63.25)
  line L2 (-74, 63.25) -> (-74, 62.25)
  line L3 (-74, 62.25) -> (-69.6, 62.25)
extrude "VL53L0X chip SRL" add sketch "VL53L0X chip SRL sketch" along normal blind 2.4 from surface at 98.8 separate body makes body 34 in component "ToF SRL"
sketch "VL53L0X module SRR sketch" plane through (0, 0, 0) normal (0, 0, 1) x (1, 0, 0) in component "ToF SRR"
  line L0 (-80.8, -57.75) -> (-80.8, -62.25)
  line L1 (-80.8, -62.25) -> (-62.8, -62.25)
  line L2 (-62.8, -62.25) -> (-62.8, -57.75)
  line L3 (-62.8, -57.75) -> (-80.8, -57.75)
extrude "VL53L0X module SRR" add sketch "VL53L0X module SRR sketch" along normal blind 21 from surface at 89.5 separate body makes body 35 in component "ToF SRR"
sketch "VL53L0X chip SRR sketch" plane through (0, 0, 0) normal (0, 0, 1) x (1, 0, 0) in component "ToF SRR"
  line L0 (-74, -62.25) -> (-74, -63.25)
  line L1 (-74, -63.25) -> (-69.6, -63.25)
  line L2 (-69.6, -63.25) -> (-69.6, -62.25)
  line L3 (-69.6, -62.25) -> (-74, -62.25)
extrude "VL53L0X chip SRR" add sketch "VL53L0X chip SRR sketch" along normal blind 2.4 from surface at 98.8 separate body makes body 36 in component "ToF SRR"
sketch "VL53L0X module RL sketch" plane through (0, 0, 0) normal (0, 0, 1) x (1, 0, 0) in component "ToF RL"
  line L0 (-81.75, 54) -> (-86.25, 54)
  line L1 (-86.25, 54) -> (-86.25, 36)
  line L2 (-86.25, 36) -> (-81.75, 36)
  line L3 (-81.75, 36) -> (-81.75, 54)
extrude "VL53L0X module RL" add sketch "VL53L0X module RL sketch" along normal blind 21 from surface at 89.5 separate body makes body 37 in component "ToF RL"
sketch "VL53L0X chip RL sketch" plane through (0, 0, 0) normal (0, 0, 1) x (1, 0, 0) in component "ToF RL"
  line L0 (-86.25, 47.2) -> (-87.25, 47.2)
  line L1 (-87.25, 47.2) -> (-87.25, 42.8)
  line L2 (-87.25, 42.8) -> (-86.25, 42.8)
  line L3 (-86.25, 42.8) -> (-86.25, 47.2)
extrude "VL53L0X chip RL" add sketch "VL53L0X chip RL sketch" along normal blind 2.4 from surface at 98.8 separate body makes body 38 in component "ToF RL"
sketch "VL53L0X module RR sketch" plane through (0, 0, 0) normal (0, 0, 1) x (1, 0, 0) in component "ToF RR"
  line L0 (-81.75, -36) -> (-86.25, -36)
  line L1 (-86.25, -36) -> (-86.25, -54)
  line L2 (-86.25, -54) -> (-81.75, -54)
  line L3 (-81.75, -54) -> (-81.75, -36)
extrude "VL53L0X module RR" add sketch "VL53L0X module RR sketch" along normal blind 21 from surface at 89.5 separate body makes body 39 in component "ToF RR"
sketch "VL53L0X chip RR sketch" plane through (0, 0, 0) normal (0, 0, 1) x (1, 0, 0) in component "ToF RR"
  line L0 (-86.25, -42.8) -> (-87.25, -42.8)
  line L1 (-87.25, -42.8) -> (-87.25, -47.2)
  line L2 (-87.25, -47.2) -> (-86.25, -47.2)
  line L3 (-86.25, -47.2) -> (-86.25, -42.8)
extrude "VL53L0X chip RR" add sketch "VL53L0X chip RR sketch" along normal blind 2.4 from surface at 98.8 separate body makes body 40 in component "ToF RR"
sketch "Lens block L sketch" plane through (0, 0, 0) normal (0, 0, 1) x (1, 0, 0) in component "Camera L"
  line L0 (-10, -10) -> (10, -10)
  line L1 (10, -10) -> (10, 10)
  line L2 (10, 10) -> (-10, 10)
  line L3 (-10, 10) -> (-10, -10)
extrude "Lens block L" add sketch "Lens block L sketch" along normal blind 23 separate body makes body 41 in component "Camera L"
sketch "Lens holder L sketch" plane through (0, 0, 0) normal (0, 0, 1) x (1, 0, 0) in component "Camera L"
  line L0 (-10, -10) -> (10, -10)
  line L1 (10, -10) -> (10, 10)
  line L2 (10, 10) -> (-10, 10)
  line L3 (-10, 10) -> (-10, -10)
extrude "Lens holder L" add sketch "Lens holder L sketch" along normal blind 2 from surface at 23 bodies 41 in component "Camera L"
sketch "OpenMV H7 Plus board L sketch" plane through (0, 0, 0) normal (0, 0, 1) x (1, 0, 0) in component "Camera L"
  line L0 (-22.5, -18) -> (22.5, -18)
  line L1 (22.5, -18) -> (22.5, 18)
  line L2 (22.5, 18) -> (-22.5, 18)
  line L3 (-22.5, 18) -> (-22.5, -18)
extrude "OpenMV H7 Plus board L" add sketch "OpenMV H7 Plus board L sketch" along normal blind 6 from surface at 25 separate body makes body 42 in component "Camera L"
sketch "Lens block R sketch" plane through (0, 0, 0) normal (0, 0, 1) x (1, 0, 0) in component "Camera R"
  line L0 (-10, -10) -> (10, -10)
  line L1 (10, -10) -> (10, 10)
  line L2 (10, 10) -> (-10, 10)
  line L3 (-10, 10) -> (-10, -10)
extrude "Lens block R" add sketch "Lens block R sketch" along normal blind 23 separate body makes body 43 in component "Camera R"
sketch "Lens holder R sketch" plane through (0, 0, 0) normal (0, 0, 1) x (1, 0, 0) in component "Camera R"
  line L0 (-10, -10) -> (10, -10)
  line L1 (10, -10) -> (10, 10)
  line L2 (10, 10) -> (-10, 10)
  line L3 (-10, 10) -> (-10, -10)
extrude "Lens holder R" add sketch "Lens holder R sketch" along normal blind 2 from surface at 23 bodies 43 in component "Camera R"
sketch "OpenMV H7 Plus board R sketch" plane through (0, 0, 0) normal (0, 0, 1) x (1, 0, 0) in component "Camera R"
  line L0 (-22.5, -18) -> (22.5, -18)
  line L1 (22.5, -18) -> (22.5, 18)
  line L2 (22.5, 18) -> (-22.5, 18)
  line L3 (-22.5, 18) -> (-22.5, -18)
extrude "OpenMV H7 Plus board R" add sketch "OpenMV H7 Plus board R sketch" along normal blind 6 from surface at 25 separate body makes body 44 in component "Camera R"
sketch "Lid sketch" plane through (0, 0, 0) normal (0, 0, 1) x (1, 0, 0) in component "Lid"
  circle A0 centre (0, 0) radius 105
extrude "Lid" add sketch "Lid sketch" along normal blind 3 from surface at 112 separate body makes body 45 in component "Lid"
sketch "Camera hump sketch" plane through (0, 0, 0) normal (0, 0, 1) x (1, 0, 0) in component "Lid"
  line L0 (-21.9288, 53) -> (28.0712, 53)
  line L1 (28.0712, 53) -> (28.0712, 93)
  line L2 (28.0712, 93) -> (-21.9288, 93)
  line L3 (-21.9288, 93) -> (-21.9288, 53)
extrude "Camera hump" add sketch "Camera hump sketch" along normal blind 8.5 from surface at 114.5 bodies 45 in component "Lid"
sketch "Camera hump sketch (1)" plane through (0, 0, 0) normal (0, 0, 1) x (1, 0, 0) in component "Lid"
  line L0 (-21.9288, -93) -> (28.0712, -93)
  line L1 (28.0712, -93) -> (28.0712, -53)
  line L2 (28.0712, -53) -> (-21.9288, -53)
  line L3 (-21.9288, -53) -> (-21.9288, -93)
extrude "Camera hump (1)" add sketch "Camera hump sketch (1)" along normal blind 8.5 from surface at 114.5 bodies 45 in component "Lid"
sketch "Camera pocket sketch" plane through (0, 0, 0) normal (0, 0, 1) x (1, 0, 0) in component "Lid"
  line L0 (-19.9288, 55) -> (26.0712, 55)
  line L1 (26.0712, 55) -> (26.0712, 91)
  line L2 (26.0712, 91) -> (-19.9288, 91)
  line L3 (-19.9288, 91) -> (-19.9288, 55)
extrude "Camera pocket" cut sketch "Camera pocket sketch" along normal blind 10 from surface at 111 bodies 45 in component "Lid"
sketch "Handle notch sketch" plane through (0, 0, 0) normal (0, 0, 1) x (1, 0, 0) in component "Lid"
  circle A0 centre (-45, 90.4) radius 5.5
extrude "Handle notch" cut sketch "Handle notch sketch" along normal blind 5 from surface at 111 bodies 45 in component "Lid"
sketch "Camera pocket sketch (1)" plane through (0, 0, 0) normal (0, 0, 1) x (1, 0, 0) in component "Lid"
  line L0 (-19.9288, -91) -> (26.0712, -91)
  line L1 (26.0712, -91) -> (26.0712, -55)
  line L2 (26.0712, -55) -> (-19.9288, -55)
  line L3 (-19.9288, -55) -> (-19.9288, -91)
extrude "Camera pocket (1)" cut sketch "Camera pocket sketch (1)" along normal blind 10 from surface at 111 bodies 45 in component "Lid"
sketch "Handle notch sketch (1)" plane through (0, 0, 0) normal (0, 0, 1) x (1, 0, 0) in component "Lid"
  circle A0 centre (-45, -90.4) radius 5.5
extrude "Handle notch (1)" cut sketch "Handle notch sketch (1)" along normal blind 5 from surface at 111 bodies 45 in component "Lid"
sketch "Start button sketch" plane through (0, 0, 0) normal (0, 0, 1) x (1, 0, 0) in component "Start button"
  circle A0 centre (-70, 0) radius 9
extrude "Start button" add sketch "Start button sketch" along normal blind 5 from surface at 115 separate body makes body 46 in component "Start button"
sketch "Victim LED sketch" plane through (0, 0, 0) normal (0, 0, 1) x (1, 0, 0) in component "Victim LED"
  circle A0 centre (-70, -30) radius 3.5
extrude "Victim LED" add sketch "Victim LED sketch" along normal blind 3.5 from surface at 115 separate body makes body 47 in component "Victim LED"
sketch "Dropper floor sketch" plane through (0, 0, 0) normal (0, 0, 1) x (1, 0, 0) in component "Dropper floor"
  circle A0 centre (-20, 0) radius 51.1342
extrude "Dropper floor" add sketch "Dropper floor sketch" along normal blind 3 from surface at 87 separate body makes body 48 in component "Dropper floor"
sketch "Slot A sketch" plane through (0, 0, 0) normal (0, 0, 1) x (1, 0, 0) in component "Dropper floor"
  line L0 (-47.2943, -37.5474) -> (-37.0413, -27.2943)
  line L1 (-37.0413, -27.2943) -> (-47.2943, -17.0413)
  line L2 (-47.2943, -17.0413) -> (-57.5474, -27.2943)
  line L3 (-57.5474, -27.2943) -> (-47.2943, -37.5474)
extrude "Slot A" cut sketch "Slot A sketch" along normal blind 5 from surface at 86 bodies 48 in component "Dropper floor"
sketch "Slot B sketch" plane through (0, 0, 0) normal (0, 0, 1) x (1, 0, 0) in component "Dropper floor"
  line L0 (-47.2943, 17.0413) -> (-37.0413, 27.2943)
  line L1 (-37.0413, 27.2943) -> (-47.2943, 37.5474)
  line L2 (-47.2943, 37.5474) -> (-57.5474, 27.2943)
  line L3 (-57.5474, 27.2943) -> (-47.2943, 17.0413)
extrude "Slot B" cut sketch "Slot B sketch" along normal blind 5 from surface at 86 bodies 48 in component "Dropper floor"
sketch "Shaft hole sketch" plane through (0, 0, 0) normal (0, 0, 1) x (1, 0, 0) in component "Dropper floor"
  circle A0 centre (-20, 0) radius 2
extrude "Shaft hole" cut sketch "Shaft hole sketch" along normal blind 5 from surface at 86 bodies 48 in component "Dropper floor"
sketch "Dropper plate sketch" plane through (0, 0, 0) normal (0, 0, 1) x (1, 0, 0) in component "Dropper plate"
  circle A0 centre (-20, 0) radius 49.1342
extrude "Dropper plate" add sketch "Dropper plate sketch" along normal blind 12 from surface at 90 separate body makes body 49 in component "Dropper plate"
sketch "Pocket 1 sketch" plane through (0, 0, 0) normal (0, 0, 1) x (1, 0, 0) in component "Dropper plate"
  line L0 (-34.9402, -28.7115) -> (-38.5636, -42.2345)
  line L1 (-38.5636, -42.2345) -> (-25.0407, -45.858)
  line L2 (-25.0407, -45.858) -> (-21.4172, -32.335)
  line L3 (-21.4172, -32.335) -> (-34.9402, -28.7115)
extrude "Pocket 1" cut sketch "Pocket 1 sketch" along normal blind 14 from surface at 89 bodies 49 in component "Dropper plate"
sketch "Pocket 2 sketch" plane through (0, 0, 0) normal (0, 0, 1) x (1, 0, 0) in component "Dropper plate"
  line L0 (-18.5828, -32.335) -> (-14.9593, -45.858)
  line L1 (-14.9593, -45.858) -> (-1.4364, -42.2345)
  line L2 (-1.4364, -42.2345) -> (-5.0598, -28.7115)
  line L3 (-5.0598, -28.7115) -> (-18.5828, -32.335)
extrude "Pocket 2" cut sketch "Pocket 2 sketch" along normal blind 14 from surface at 89 bodies 49 in component "Dropper plate"
sketch "Pocket 3 sketch" plane through (0, 0, 0) normal (0, 0, 1) x (1, 0, 0) in component "Dropper plate"
  line L0 (-2.6052, -27.2943) -> (7.2943, -37.1938)
  line L1 (7.2943, -37.1938) -> (17.1938, -27.2943)
  line L2 (17.1938, -27.2943) -> (7.2943, -17.3948)
  line L3 (7.2943, -17.3948) -> (-2.6052, -27.2943)
extrude "Pocket 3" cut sketch "Pocket 3 sketch" along normal blind 14 from surface at 89 bodies 49 in component "Dropper plate"
sketch "Pocket 4 sketch" plane through (0, 0, 0) normal (0, 0, 1) x (1, 0, 0) in component "Dropper plate"
  line L0 (8.7115, -14.9402) -> (22.2345, -18.5636)
  line L1 (22.2345, -18.5636) -> (25.858, -5.0407)
  line L2 (25.858, -5.0407) -> (12.335, -1.4172)
  line L3 (12.335, -1.4172) -> (8.7115, -14.9402)
extrude "Pocket 4" cut sketch "Pocket 4 sketch" along normal blind 14 from surface at 89 bodies 49 in component "Dropper plate"